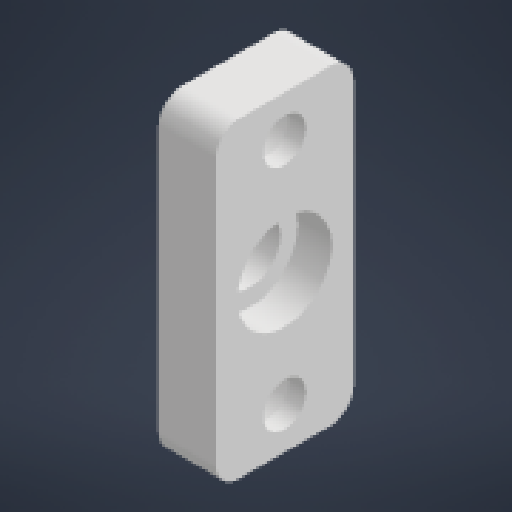
# Autodesk Inventor part: PCB_Housing_07_V4
Saved by Autodesk Inventor 2026.2 (Build 302298000, 298)
## iProperties
Created: 2026-03-17
Part Number: PCB_Housing_07_V4
Material: Generic
Document SubType Name: Modeling
Designer: vckot
Density: 1 g/cm^3
Appearance: Default
Author: vckot
Autodesk Inventor part; units mm, degrees
ref_plane "YZ Plane" through (0, 0, 0) normal (1, 0, 0) x (0, 1, 0)
ref_plane "XZ Plane" through (0, 0, 0) normal (0, 1, 0) x (-1, 0, 0)
ref_plane "XY Plane" through (0, 0, 0) normal (0, 0, 1) x (1, 0, 0)
sketch "Sketch1" plane through (0, 0, 0) normal (1, 0, 0) x (0, 1, 0)
  circle A0 centre (0, 0) radius 4.125
  circle A1 centre (-10, 0) radius 2.25
  circle A2 centre (10, 0) radius 2.25
  line L0 (-14.125, 6) -> (-14.125, -6)
  line L1 (14.125, 6) -> (14.125, -6)
  line L2 (-14.125, -6) -> (14.125, -6)
  line L3 (14.125, 6) -> (-14.125, 6)
  point P0 (-10, 4.125)
  point P1 (0, 4.125)
  point P2 (10, 4.125)
  point P3 (0, 4.125)
  dimension "d0" = 8.25
  dimension "d1" = 4.5
  dimension "d2" = 4.5
  dimension "d3" = 10
  dimension "d4" = 10
  dimension "d28" = 12
  dimension "d29" = 6
  dimension "d30" = 14.125
  dimension "d31" = 28.25
  constraints: 8 end point, 3 centre point, 2 coincident, 2 horizontal alignment, 2 perpendicular, 2 point on circle, 1 horizontal
  measures "d0" diameter of A0
  measures "d1" diameter of A1
  measures "d2" diameter of A2
  measures "d3" distance of A0.centre A1.centre
  measures "d4" distance of A0.centre A2.centre
  measures "d28" distance between parallel lines of L2 L3
  measures "d29" distance from line of L2 A0.centre
  measures "d30" distance from line of A0.centre L0
  measures "d31" distance between parallel lines of L1 L0
extrude "Extrusion1" add sketch "Sketch1" along normal blind 5 contours A1 | A2 | L3 L1 L2 L0
sketch "Sketch2" plane through (0, 0, 0) normal (-1, 0, 0) x (0, 0, 1)
  circle A0 centre (0, 0) radius 2.625
  circle A1 centre (0, 0) radius 4.125 projected
  circle A2 centre (0, 10) radius 2.25 projected
  circle A3 centre (0, -10) radius 2.25 projected
  point P0 (4.125, 0)
  dimension "d13" = 5.25
  constraints: 1 centre point, 1 coincident, 1 horizontal alignment
  measures "d13" diameter of A0
extrude "Extrusion2" add sketch "Sketch1" along normal blind 2 contours A0
extrude "Extrusion3" cut sketch "Sketch2" against normal blind 2 contours A0
hole "Hole1" at (0, 10, 0) at (0, -10, 0) direction (1, 0, 0) diameter 3.75 depth 8 tip angle 118 counterbore diameter 6 counterbore depth 3.5
thicken "Thicken1" operation add thickness 0.5 both sides no extend neighbours yes toward (0, 1, 0) faces at (1.6667, -14.125, 2)
thicken "Thicken2" operation add thickness 0.5 both sides no extend neighbours yes toward (0, -1, 0) faces at (1.6667, 14.125, -2)
fillet "Fillet1" radius 2 4 edges at (2.5, 13.625, -6) (2.5, 13.625, 6) (2.5, -13.625, 6) (2.5, -13.625, -6)
body "Solid1"
